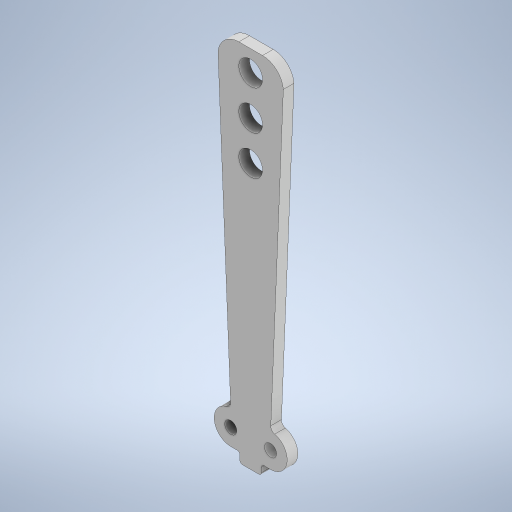
# Autodesk Inventor part: Blade
Saved by Autodesk Inventor 2023.5 (Build 275446000, 446)
## iProperties
Created: 2025-04-03
Part Number: Blade
Material: Generic
Document SubType Name: Modeling
Designer: huy20
Density: 1 g/cm^3
Appearance: Default
Author: huy20
Autodesk Inventor part; units mm, degrees
ref_plane "YZ Plane" through (0, 0, 0) normal (1, 0, 0) x (0, 1, 0)
ref_plane "XZ Plane" through (0, 0, 0) normal (0, 1, 0) x (-1, 0, 0)
ref_plane "XY Plane" through (0, 0, 0) normal (0, 0, 1) x (1, 0, 0)
sketch "Sketch1" plane through (0, 0, 0) normal (0, 0, 1) x (1, 0, 0)
  line L0 (12.4954, 128.3185) -> (7.6936, 14.3066)
  circle A0 centre (-7.62, 6.2119) radius 2.286
  line L1 (7.62, 8.4979) -> (7.9776, 8.4697)
  line L2 (7.2624, 3.954) -> (7.62, 3.9259)
  circle A1 centre (7.62, 6.2119) radius 2.286
  arc A2 (-9.1979, 12.3627) -> (-7.62, -0.1381) centre (-7.62, 6.2119) ccw
  arc A3 (7.62, -0.1381) -> (9.198, 12.3626) centre (7.62, 6.2119) ccw
  line L3 (-7.6934, 14.3065) -> (-12.4926, 128.3185)
  arc A4 (-4.1275, -2.9481) -> (-3.1275, -3.9481) centre (-3.1275, -2.9481) ccw
  arc A5 (3.1275, -3.9481) -> (4.1275, -2.9481) centre (3.1275, -2.9481) ccw
  line L4 (7.62, -0.1381) -> (5.1275, -0.1381)
  line L5 (-5.1275, -0.1381) -> (-7.62, -0.1381)
  arc A6 (-4.1275, -1.1381) -> (-5.1275, -0.1381) centre (-5.1275, -1.1381) ccw
  arc A7 (5.1275, -0.1381) -> (4.1275, -1.1381) centre (5.1275, -1.1381) ccw
  arc A8 (7.6968, 14.3841) -> (9.198, 12.3626) centre (9.6951, 14.2999) ccw
  arc A9 (-9.1979, 12.3627) -> (-7.6966, 14.3841) centre (-9.6949, 14.3) ccw
  line L6 (12.4954, 128.3185) -> (12.4954, 135.5817)
  line L7 (12.4954, 135.5817) -> (-12.4926, 135.5817)
  line L8 (-12.4926, 135.5817) -> (-12.4926, 128.3185)
  line L9 (-4.1275, -1.1381) -> (-4.1275, -2.9481)
  line L10 (-3.1275, -3.9481) -> (3.1275, -3.9481)
  line L11 (4.1275, -1.1381) -> (4.1275, -2.9481)
  point P0 (-5.1275, -0.1381)
  point P1 (0.0014, 135.5817)
  point P2 (0, 0)
  dimension "d2" = 15.24
  dimension "d15" = 4.572
  dimension "d16" = 24.988
  dimension "d17" = 4.822
  dimension "d74" = 10.16
  dimension "d75" = 3.9482
  dimension "d122" = 2
  constraints: 24 end point, 18 point on circle, 15 tangent, 10 centre point, 6 equal radius, 6 point on line, 4 parallel, 3 coincident, 2 horizontal, 2 vertical, 1 collinear, 1 midpoint
  measures "d2" distance of A1.centre point (-7.62, 6.212)
  measures "d15" diameter of A0
  measures "d16" distance of L6.end L7.end
  measures "d17" angle of L3 L0
  measures "d74" distance from line of L10 A1.centre
  measures "d75" distance from line of L10 point (0, 0)
  measures "d122" radius of A8
extrude "Extrusion1" add sketch "Sketch1" along normal mid plane 4.077
fillet "Fillet1" radius 8 2 edges at (12.4954, 135.5817, 0) (-12.4926, 135.5817, 0)
sketch "Sketch2" plane through (0, 0, 2.0385) normal (0, 0, 1) x (1, 0, 0)
  arc A0 (-4.5266, 135.5817) -> (-12.4926, 128.3185) centre (-4.5266, 127.5817) ccw projected
  line L0 (-12.4926, 128.3185) -> (-7.6966, 14.3841) projected
  arc A1 (-9.1979, 12.3627) -> (-7.6966, 14.3841) centre (-9.6949, 14.3) ccw projected
  arc A2 (-9.1979, 12.3627) -> (-7.62, -0.1381) centre (-7.62, 6.2119) ccw projected
  line L1 (-7.62, -0.1381) -> (-5.1275, -0.1381) projected
  arc A3 (-4.1275, -1.1381) -> (-5.1275, -0.1381) centre (-5.1275, -1.1381) ccw projected
  line L2 (-4.1275, -1.1381) -> (-4.1275, -2.9481) projected
  arc A4 (-4.1275, -2.9481) -> (-3.1275, -3.9481) centre (-3.1275, -2.9481) ccw projected
  line L3 (-3.1275, -3.9481) -> (3.1275, -3.9481) projected
  arc A5 (3.1275, -3.9481) -> (4.1275, -2.9481) centre (3.1275, -2.9481) ccw projected
  line L4 (4.1275, -2.9481) -> (4.1275, -1.1381) projected
  arc A6 (5.1275, -0.1381) -> (4.1275, -1.1381) centre (5.1275, -1.1381) ccw projected
  line L5 (5.1275, -0.1381) -> (7.62, -0.1381) projected
  arc A7 (7.62, -0.1381) -> (9.198, 12.3626) centre (7.62, 6.2119) ccw projected
  arc A8 (7.6968, 14.3841) -> (9.198, 12.3626) centre (9.6951, 14.2999) ccw projected
  line L6 (7.6968, 14.3841) -> (12.4954, 128.3185) projected
  arc A9 (12.4954, 128.3185) -> (4.5294, 135.5817) centre (4.5294, 127.5817) ccw projected
  line L7 (4.5294, 135.5817) -> (-4.5266, 135.5817) projected
  circle A10 centre (-7.62, 6.2119) radius 2.286 projected
  circle A11 centre (7.62, 6.2119) radius 2.286 projected
  line L8 (-4.5266, 127.5817) -> (4.5294, 127.5817)
  circle A12 centre (0.0014, 127.5817) radius 4.528
  circle A13 centre (0.0014, 112.5817) radius 4.528
  circle A14 centre (0.0014, 97.5817) radius 4.528
  point P0 (0, 0)
  dimension "d114" = 15
  dimension "d115" = 15
  dimension "d118" = 23
  dimension "d119" = 38
  constraints: 2 centre point, 2 end point, 1 horizontal, 1 horizontal alignment, 1 midpoint, 4 other
  measures "d114" distance of A13.centre point (0.001, 127.582)
  measures "d115" distance of A14.centre A13.centre
  measures "d118" distance from line of L7 A13.centre
  measures "d119" distance from line of A14.centre L7
extrude "Extrusion2" cut sketch "Sketch2" against normal through all contours A12 L8 | L8 A12 | A13 | A14
body "Solid1"
